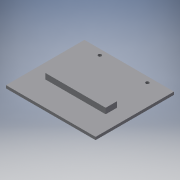
# Autodesk Inventor part: mainboard
Saved by Autodesk Inventor 2018 (Build 220112000, 112)
## iProperties
Created: 2017-12-03
Part Number: mainboard
Material: Generic
Document SubType Name: Modeling
Designer: Cole Tucker
Density: 1 g/cm^3
Appearance: Default
Author: Cole Tucker
Autodesk Inventor part; units mm, degrees
ref_plane "YZ Plane" through (0, 0, 0) normal (1, 0, 0) x (0, 1, 0)
ref_plane "XZ Plane" through (0, 0, 0) normal (0, 1, 0) x (-1, 0, 0)
ref_plane "XY Plane" through (0, 0, 0) normal (0, 0, 1) x (1, 0, 0)
sketch "Sketch1" plane through (0, 0, 0) normal (0, 1, 0) x (-1, 0, 0)
  line L0 (0, 0) -> (-101.6, 0)
  line L1 (-101.6, 0) -> (-101.6, -88.9)
  line L2 (-101.6, -88.9) -> (0, -88.9)
  line L3 (0, -88.9) -> (0, 0)
  line L4 (-50.8, -88.9) -> (-23.8125, -88.9)
  line L5 (-50.8, -88.9) -> (-77.7875, -88.9)
  line L6 (-77.7875, -88.9) -> (-77.7875, -82.55)
  line L7 (-23.8125, -88.9) -> (-23.8125, -82.55)
  circle A0 centre (-23.8125, -82.55) radius 1.905
  circle A1 centre (-77.7875, -82.55) radius 1.905
  dimension "d0" = 101.6
  dimension "d1" = 88.9
  dimension "d2" = 26.9875
  dimension "d3" = 26.9875
  dimension "d4" = 6.35
  dimension "d5" = 6.35
  dimension "d6" = 3.81
  dimension "d7" = 3.81
  constraints: 16 end point, 2 centre point, 2 coincident, 2 parallel, 2 perpendicular, 2 point on line, 1 horizontal, 1 midpoint, 1 vertical
  measures "d0" distance of L2.end L1.end
  measures "d1" distance of L1.end L0.end
  measures "d2" distance of L4.start L4.end
  measures "d3" distance of L4.start L5.end
  measures "d4" distance of L5.end L6.end
  measures "d5" distance of L4.end L7.end
  measures "d6" diameter of A0
  measures "d7" diameter of A1
extrude "Extrusion1" add sketch "Sketch1" along normal blind 3.175
sketch "Sketch2" plane through (0, 0, 0) normal (0, -1, 0) x (1, 0, 0)
  line L0 (101.6, -88.9) -> (0, -88.9) projected
  line L1 (50.8, -88.9) -> (50.8, -12.7)
  line L2 (50.8, -12.7) -> (76.2, -12.7)
  line L3 (76.2, -12.7) -> (25.4, -12.7)
  line L4 (25.4, -12.7) -> (25.4, -6.35)
  line L5 (25.4, -6.35) -> (76.2, -6.35)
  line L6 (76.2, -6.35) -> (76.2, -12.7)
  point P0 (0, 0)
  dimension "d10" = 76.2
  dimension "d11" = 25.4
  dimension "d12" = 50.8
  dimension "d13" = 6.35
  constraints: 12 end point, 2 parallel, 2 perpendicular, 1 horizontal, 1 midpoint, 1 vertical
  measures "d10" distance of L1.start L1.end
  measures "d11" distance of L1.end L2.end
  measures "d12" distance of L4.end L5.end
  measures "d13" distance of L3.end L4.end
extrude "Extrusion2" add sketch "Sketch2" along normal blind 6.35
sketch "Sketch3" plane through (0, 3.175, 0) normal (0, 1, 0) x (1, 0, 0)
  line L0 (0, 0) -> (101.6, 0) projected
  line L1 (0, 0) -> (0, 34.29)
  line L2 (0, 88.9) -> (0, 0) projected
  line L3 (0, 34.29) -> (50.8, 34.29)
  line L4 (50.8, 34.29) -> (50.8, 40.64)
  line L5 (50.8, 40.64) -> (16.51, 40.64)
  line L6 (16.51, 40.64) -> (85.09, 40.64)
  line L7 (85.09, 40.64) -> (85.09, 27.94)
  line L8 (85.09, 27.94) -> (16.51, 27.94)
  line L9 (16.51, 27.94) -> (16.51, 40.64)
  dimension "d16" = 34.29
  dimension "d17" = 50.8
  dimension "d18" = 6.35
  dimension "d19" = 34.29
  dimension "d20" = 68.58
  dimension "d21" = 12.7
  constraints: 16 end point, 3 horizontal, 2 parallel, 2 perpendicular, 1 point on line
  measures "d16" distance of L0.start L1.end
  measures "d17" distance of L1.end L3.end
  measures "d18" distance of L3.end L4.end
  measures "d19" distance of L4.end L5.end
  measures "d20" distance of L7.end L8.end
  measures "d21" distance of L6.end L7.end
extrude "Extrusion3" add sketch "Sketch3" along normal blind 6.35
body "Solid1"
